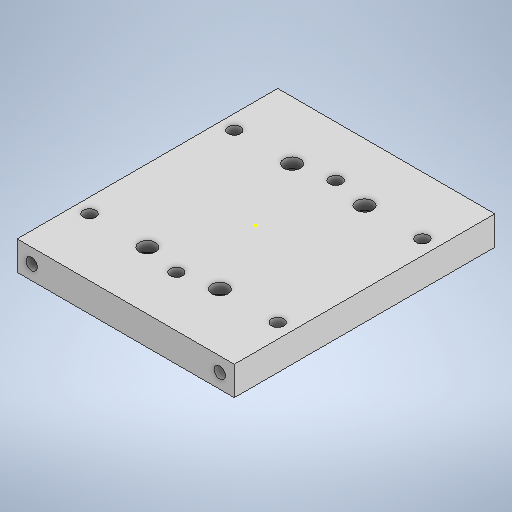
# Autodesk Inventor part: Rb PEEK - Arriba
Saved by Autodesk Inventor 2025.3 (Build 293356000, 356)
## iProperties
Created: 2025-05-09
Part Number: Rb PEEK - Arriba
Material: Generic
Document SubType Name: Modeling
Designer: E. Moreno
Density: 1 g/cm^3
Appearance: Default
Title: Rb PEEK - Abajo
Author: E. Moreno
Autodesk Inventor part; units mm, degrees
ref_plane "YZ Plane" through (0, 0, 0) normal (1, 0, 0) x (0, 1, 0)
ref_plane "XZ Plane" through (0, 0, 0) normal (0, 1, 0) x (-1, 0, 0)
ref_plane "XY Plane" through (0, 0, 0) normal (0, 0, 1) x (1, 0, 0)
sketch "Sketch1" plane through (0, 0, 0) normal (0, 1, 0) x (-1, 0, 0)
  line L0 (-37.5, 45) -> (37.5, 45)
  line L1 (37.5, 45) -> (37.5, -45)
  line L2 (37.5, -45) -> (-37.5, -45)
  line L3 (-37.5, -45) -> (-37.5, 45)
  line L4 (-37.5, 45) -> (37.5, -45) construction
  line L5 (37.5, 45) -> (-37.5, -45) construction
  point P0 (0, 0)
  dimension "d0" = 75
  dimension "d1" = 90
  constraints: 12 end point, 2 midpoint, 2 parallel, 1 horizontal, 1 perpendicular
  measures "d0" distance of L1.end L2.end
  measures "d1" distance of L0.end L1.end
extrude "Extrusion1" add sketch "Sketch1" along normal blind 10
sketch "Sketch2" plane through (0, 10, 0) normal (0, 1, 0) x (1, 0, 0)
  line L0 (-37.5, -45) -> (37.5, -45) projected
  line L1 (37.5, -45) -> (37.5, -25)
  line L2 (37.5, -45) -> (37.5, 45) projected
  line L3 (37.5, -25) -> (32.5, -25)
  circle A0 centre (32.5, -25) radius 2.15
  line L4 (0, 0) -> (37.5, 0)
  line L5 (-37.5, 45) -> (37.5, 45)
  line L6 (37.5, 45) -> (37.5, 25)
  line L7 (37.5, 45) -> (37.5, -45)
  line L8 (37.5, 25) -> (32.5, 25)
  circle A1 centre (32.5, 25) radius 2.15
  line L9 (0, -45) -> (0, 45)
  line L10 (-37.5, -45) -> (-37.5, -25)
  line L11 (-37.5, -45) -> (-37.5, 45)
  line L12 (-37.5, -25) -> (-32.5, -25)
  circle A2 centre (-32.5, -25) radius 2.15
  line L13 (-37.5, 45) -> (-37.5, 25)
  line L14 (-37.5, 45) -> (-37.5, -45)
  line L15 (-37.5, 25) -> (-32.5, 25)
  circle A3 centre (-32.5, 25) radius 2.15
  point P0 (-37.5, 0)
  dimension "d4" = 20
  dimension "d5" = 5
  dimension "d6" = 4.3
  constraints: 28 end point, 17 symmetric about line, 4 centre point, 4 coincident, 4 point on line, 3 midpoint, 1 horizontal, 3 other
  measures "d4" distance of L0.end L1.end
  measures "d5" distance of L1.end L3.end
  measures "d6" diameter of A0
extrude "Extrusion2" cut sketch "Sketch2" against normal blind 10 contours A0 | A1 | A2 | A3
sketch "Sketch3" plane through (0, 10, 0) normal (0, 1, 0) x (1, 0, 0)
  circle A0 centre (32.5, -25) radius 3.61
  circle A1 centre (32.5, -25) radius 2.15 projected
  line L0 (0, 0) -> (29.9913, 0)
  line L1 (-37.5, -45) -> (37.5, -45) projected
  line L2 (0, -45) -> (0, 45)
  circle A2 centre (32.5, -25) radius 2
  circle A3 centre (32.5, 25) radius 3.61
  circle A4 centre (32.5, 25) radius 2.15
  circle A5 centre (32.5, 25) radius 2
  circle A6 centre (-32.5, -25) radius 3.61
  circle A7 centre (-32.5, -25) radius 2.15
  circle A8 centre (-32.5, -25) radius 2
  circle A9 centre (-32.5, 25) radius 3.61
  circle A10 centre (-32.5, 25) radius 2.15
  circle A11 centre (-32.5, 25) radius 2
  point P0 (22.5, -40)
  point P1 (-29.9913, 0)
  dimension "d11" = 7.22
  dimension "d14" = 4
  constraints: 11 centre point, 10 symmetric about line, 4 end point, 2 concentric, 1 horizontal, 1 midpoint, 9 other
  measures "d11" diameter of A0
  measures "d14" diameter of A2
extrude "Extrusion3" cut sketch "Sketch3" against normal blind 4.5 contours A0 | A3 | A6 | A9
mirror "Mirror1" about plane through (0, 0, 0) normal (0, 1, 0) remove original yes
sketch "Boceto12" plane through (-37.5, 0, -45) normal (0, 1, 0) x (1, 0, 0)
  point P0 (37.5, -45)
sketch "Boceto13" plane through (-37.5, -10, -45) normal (0, -1, 0) x (1, 0, 0)
  line L0 (37.5, 45) -> (37.5, 17.5)
  circle A0 centre (37.5, 17.5) radius 2.15
  line L1 (37.5, 45) -> (37.5, 72.5)
  circle A1 centre (37.5, 72.5) radius 2.15
  dimension "d69" = 27.5
  dimension "d70" = 4.3
  dimension "d71" = 27.5
  dimension "d72" = 4.3
  constraints: 4 end point, 2 centre point, 2 coincident, 2 vertical
  measures "d69" distance of L0.start L0.end
  measures "d70" diameter of A0
  measures "d71" distance of L0.start L1.end
  measures "d72" diameter of A1
extrude "Extrusión12" cut sketch "Boceto13" against normal blind 10
sketch "Boceto14" plane through (-37.5, -10, -45) normal (0, -1, 0) x (1, 0, 0)
  circle A0 centre (37.5, 72.5) radius 3.61
  circle A1 centre (37.5, 17.5) radius 3.61
  circle A2 centre (37.5, 72.5) radius 2.15 projected
  circle A3 centre (37.5, 17.5) radius 2.15 projected
  point P0 (37.5, 45)
  dimension "d75" = 7.22
  dimension "d76" = 7.22
  constraints: 2 centre point, 2 concentric
  measures "d75" diameter of A0
  measures "d76" diameter of A1
extrude "Extrusión13" cut sketch "Boceto14" against normal blind 4.5 contours A0 | A1 | A2
sketch "Sketch15" plane through (37.5, 0, -45) normal (0, 0, -1) x (-1, 0, 0)
  line L0 (0, 0) -> (0, -10) projected
  line L1 (0, -5) -> (5, -5)
  circle A0 centre (5, -5) radius 2
  line L2 (75, 0) -> (75, -10) projected
  line L3 (75, -5) -> (70, -5)
  circle A1 centre (70, -5) radius 2
  point P0 (37.5, 0)
  dimension "d80" = 5
  dimension "d81" = 4
  dimension "d82" = 5
  dimension "d83" = 4
  constraints: 4 end point, 2 centre point, 2 coincident, 2 horizontal, 2 midpoint
  measures "d80" distance of L1.start L1.end
  measures "d81" diameter of A0
  measures "d82" distance of L3.start L3.end
  measures "d83" diameter of A1
extrude "Extrusion14" cut sketch "Sketch15" against normal blind 15
sketch "Sketch16" plane through (-37.5, 0, 45) normal (0, 0, 1) x (1, 0, 0)
  line L0 (0, 0) -> (0, -10) projected
  line L1 (0, -5) -> (5, -5)
  circle A0 centre (5, -5) radius 2
  line L2 (75, 0) -> (75, -10) projected
  line L3 (75, -5) -> (70, -5)
  circle A1 centre (70, -5) radius 2
  point P0 (37.5, 0)
  dimension "d86" = 5
  dimension "d87" = 4
  dimension "d88" = 5
  dimension "d89" = 4
  constraints: 4 end point, 2 centre point, 2 coincident, 2 horizontal, 2 midpoint
  measures "d86" distance of L1.start L1.end
  measures "d87" diameter of A0
  measures "d88" distance of L3.start L3.end
  measures "d89" diameter of A1
extrude "Extrusion15" cut sketch "Sketch16" against normal blind 15
thread "Thread1" size "M4x0.7" class "6H" standard "ANSI Metric M Profile" full length
thread "Thread2" size "M4x0.7" class "6H" standard "ANSI Metric M Profile" full length
thread "Thread3" size "M4x0.7" class "6H" standard "ANSI Metric M Profile" full length
thread "Thread4" size "M4x0.7" class "6H" standard "ANSI Metric M Profile" full length
sketch "Sketch17" plane through (-37.5, 0, -45) normal (0, 1, 0) x (1, 0, 0)
  line L0 (37.5, -45) -> (37.5, -20.0064)
  line L1 (37.5, -20.0064) -> (24.9778, -20.0064)
  circle A0 centre (24.9778, -20.0064) radius 1.6
  circle A1 centre (50.0222, -20.0064) radius 1.6
  line L2 (0, 0) -> (0, -90) projected
  line L3 (0, -45) -> (75, -45)
  line L4 (75, -90) -> (75, 0) projected
  circle A2 centre (24.9778, -69.9936) radius 1.6
  circle A3 centre (50.0222, -69.9936) radius 1.6
  dimension "d100" = 24.9936
  dimension "d101" = 12.5222
  dimension "d102" = 3.2
  constraints: 6 end point, 5 symmetric about line, 4 centre point, 3 coincident, 2 midpoint, 1 horizontal, 1 vertical, 3 other
  measures "d100" distance of L0.start L0.end
  measures "d101" distance of L0.end L1.end
  measures "d102" diameter of A0
extrude "Extrusion16" cut sketch "Sketch17" against normal blind 10
sketch "Sketch18" plane through (-37.5, 0, -45) normal (0, 1, 0) x (1, 0, 0)
  circle A0 centre (24.9778, -20.0064) radius 1.6 projected
  circle A1 centre (24.9778, -20.0064) radius 2.84
  line L0 (75, 0) -> (0, 0) projected
  line L1 (37.5, 0) -> (37.5, -90)
  line L2 (0, -90) -> (75, -90) projected
  line L3 (0, 0) -> (0, -90) projected
  line L4 (0, -45) -> (75, -45)
  line L5 (75, -90) -> (75, 0) projected
  circle A2 centre (50.0222, -20.0064) radius 1.6
  circle A3 centre (50.0222, -20.0064) radius 2.84
  circle A4 centre (24.9778, -69.9936) radius 1.6
  circle A5 centre (24.9778, -69.9936) radius 2.84
  circle A6 centre (50.0222, -69.9936) radius 1.6
  circle A7 centre (50.0222, -69.9936) radius 2.84
  point P0 (37.5, -45)
  dimension "d105" = 5.68
  constraints: 7 centre point, 6 symmetric about line, 4 coincident, 4 end point, 4 midpoint, 6 other
  measures "d105" diameter of A1
extrude "Extrusion17" cut sketch "Sketch18" against normal blind 3.5 contours A1 | A3 | A5 | A7
body "Solid1"
